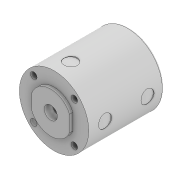
# Autodesk Inventor part: gear(49ratio)
Saved by Autodesk Inventor 2020 (Build 240168000, 168)
## iProperties
Created: 2020-08-28
Part Number: gear(49ratio)
Material: 일반
Document SubType Name: Modeling
Designer: 이호석
Mass: 65.0575 g
Surface Area: 95.0855 cm^2
Volume: 65.0575 cm^3
Density: 1 g/cm^3
Appearance: 기본값
Author: 이호석
Autodesk Inventor part; units mm, degrees
ref_plane "YZ Plane" through (0, 0, 0) normal (1, 0, 0) x (0, 1, 0)
ref_plane "XZ Plane" through (0, 0, 0) normal (0, 1, 0) x (-1, 0, 0)
ref_plane "XY Plane" through (0, 0, 0) normal (0, 0, 1) x (1, 0, 0)
sketch "스케치1" plane through (0, 0, 0) normal (0, 0, 1) x (1, 0, 0)
  circle A0 centre (0, 0) radius 21.2
  dimension "d0" = 42.4
  constraints: 1 centre point, 1 coincident
  measures "d0" diameter of A0
extrude "돌출1" add sketch "스케치1" along normal blind 45.9
sketch "스케치2" plane through (0, 0, 45.9) normal (0, 0, 1) x (1, 0, 0)
  circle A0 centre (0, 0) radius 12.5
  line L0 (-11.5, -4.899) -> (-11.5, 4.899)
  line L1 (11.5, -4.899) -> (11.5, 4.899)
  line L2 (0, 0) -> (17.5, 0) construction
  circle A1 centre (12.3744, -12.3744) radius 2
  circle A2 centre (12.3744, 12.3744) radius 2
  circle A3 centre (-12.3744, 12.3744) radius 2
  circle A4 centre (-12.3744, -12.3744) radius 2
  dimension "d5" = 360
  constraints: 6 end point, 5 centre point, 4 point on circle, 1 coincident, 1 horizontal, 9 other
extrude "돌출2" cut sketch "스케치2" against normal blind 6 contours A1 | A2 | A3 | A4
sketch "스케치3" plane through (0, 0, 45.9) normal (0, 0, 1) x (1, 0, 0)
  circle A0 centre (0, 0) radius 12.5
  line L0 (-11.5, -4.899) -> (-11.5, 4.899)
  line L1 (11.5, -4.899) -> (11.5, 4.899)
  line L2 (0, 0) -> (17.5, 0) construction
  circle A1 centre (12.3744, -12.3744) radius 2
  circle A2 centre (12.3744, 12.3744) radius 2
  circle A3 centre (-12.3744, 12.3744) radius 2
  circle A4 centre (-12.3744, -12.3744) radius 2
  dimension "d10" = 360
  constraints: 6 end point, 5 centre point, 4 point on circle, 1 coincident, 1 horizontal, 9 other
extrude "돌출3" add sketch "스케치3" along normal blind 2 contours L1 A0 L0
sketch "스케치4" plane through (0, 0, 47.9) normal (0, 0, 1) x (1, 0, 0)
  circle A0 centre (0, 0) radius 4
  dimension "d13" = 8
  constraints: 1 centre point, 1 coincident
  measures "d13" diameter of A0
extrude "돌출4" cut sketch "스케치4" against normal blind 5
ref_plane "작업 평면1" through (21.2, 0, 0) normal (1, 0, 0) x (0, 1, 0)
sketch "스케치5" plane through (21.2, 0, 0) normal (1, 0, 0) x (0, 1, 0)
  line L0 (21.2, 45.9) -> (-21.2, 45.9) projected
  line L1 (21.2, 0) -> (-21.2, 0) projected
  line L2 (-4.899, 45.9) -> (4.899, 45.9) projected
  line L3 (0, 45.9) -> (0, 35.9)
  line L4 (0, 35.9) -> (0, 10)
  circle A0 centre (0, 10) radius 4
  circle A1 centre (0, 35.9) radius 4
  point P0 (0, 0)
  dimension "d16" = 10
  dimension "d17" = 25.9
  dimension "d18" = 8
  constraints: 4 end point, 2 centre point, 2 coincident, 1 midpoint, 1 point on line, 1 vertical
  measures "d16" distance of L3.start L3.end
  measures "d17" distance of L3.end L4.end
  measures "d18" diameter of A0
extrude "돌출5" cut sketch "스케치5" against normal blind 0.5
ref_plane "작업 평면5" through (0, 21.2, 0) normal (0, 1, 0) x (-1, 0, 0)
sketch "스케치7" plane through (0, 21.2, 0) normal (0, 1, 0) x (-1, 0, 0)
  line L0 (0, 0) -> (0, 35.9)
  line L1 (-11.5, 45.9) -> (11.5, 45.9) projected
  circle A0 centre (0, 35.9) radius 4
  dimension "d28" = 35.9
  dimension "d29" = 8
  constraints: 2 end point, 1 centre point, 1 coincident, 1 perpendicular
  measures "d28" distance of L0.start L0.end
  measures "d29" diameter of A0
extrude "돌출7" cut sketch "스케치7" against normal blind 0.5
pattern_circular "원형 패턴2" count 2 over 360 about axis through (0, 0, 0) along (0, 0, 1) of "돌출5", "돌출7"
fillet "모깎기1" radius 1 1 edges at (-21.2, 0, 0)
